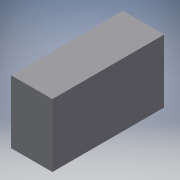
# Autodesk Inventor part: bat9V
Saved by Autodesk Inventor 2018 (Build 220112000, 112)
## iProperties
Created: 2018-07-19
Part Number: bat9V
Material: Generic
Document SubType Name: Modeling
Designer: julien.allali
Density: 1 g/cm^3
Appearance: Default
Author: julien.allali
Autodesk Inventor part; units mm, degrees
ref_plane "YZ Plane" through (0, 0, 0) normal (1, 0, 0) x (0, 1, 0)
ref_plane "XZ Plane" through (0, 0, 0) normal (0, 1, 0) x (-1, 0, 0)
ref_plane "XY Plane" through (0, 0, 0) normal (0, 0, 1) x (1, 0, 0)
sketch "Sketch1" plane through (0, 0, 0) normal (0, 1, 0) x (-1, 0, 0)
  line L0 (0, 0) -> (17, 0)
  line L1 (17, 0) -> (17, -26)
  line L2 (17, -26) -> (0, -26)
  line L3 (0, -26) -> (0, 0)
  dimension "d0" = 26
  dimension "d1" = 17
  constraints: 8 end point, 2 parallel, 1 horizontal, 1 perpendicular
  measures "d0" distance of L0.end L1.end
  measures "d1" distance between parallel lines of L3 L1
extrude "Extrusion1" add sketch "Sketch1" along normal blind 46
sketch "Sketch2" plane through (0, 46, 0) normal (0, 1, 0) x (1, 0, 0)
  line L0 (-17, 0) -> (0, 0) construction
  line L1 (-8.5, 0) -> (-8.5, 26) construction
  line L2 (0, 26) -> (-17, 26) construction
  circle A0 centre (-8.5, 20.5) radius 2.8
  line L3 (-3.9389, 6) -> (-6.2195, 2.05)
  line L4 (-6.2195, 2.05) -> (-10.7805, 2.05)
  line L5 (-10.7805, 2.05) -> (-13.0611, 6)
  line L6 (-13.0611, 6) -> (-10.7805, 9.95)
  line L7 (-10.7805, 9.95) -> (-6.2195, 9.95)
  line L8 (-6.2195, 9.95) -> (-3.9389, 6)
  point P0 (-8.5, 6)
  dimension "d5" = 7.9
  dimension "d6" = 6
  dimension "d7" = 5.5
  dimension "d8" = 5.6
  constraints: 14 end point, 2 midpoint, 2 point on line, 1 centre point, 1 parallel, 13 other
  measures "d5" distance between parallel lines of L3 L6
  measures "d6" distance from line of L0 point (-8.5, 6)
  measures "d7" distance from line of L2 A0.centre
  measures "d8" diameter of A0
extrude "Extrusion2" add sketch "Sketch2" along normal blind 2
equation "\"d2\" = height"
equation "\"height\" = 46"
body "Solid1"
